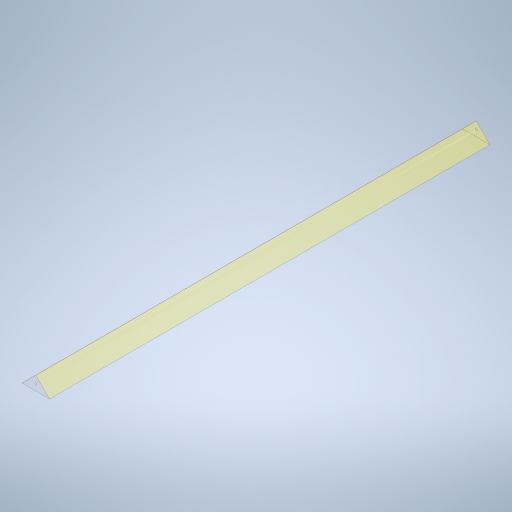
# Autodesk Inventor part: Centelladora triangular
Saved by Autodesk Inventor 2024.2 (Build 282272000, 272)
## iProperties
Created: 2024-08-22
Part Number: Centelladora triangular
Material: PMMA Plastic
Document SubType Name: Modeling
Designer: ja.restrepo1
Density: 1.188 g/cm^3
Appearance: Polycarbonate - Clear
Author: ja.restrepo1
Autodesk Inventor part; units mm, degrees
ref_plane "YZ Plane" through (0, 0, 0) normal (1, 0, 0) x (0, 1, 0)
ref_plane "XZ Plane" through (0, 0, 0) normal (0, 1, 0) x (-1, 0, 0)
ref_plane "XY Plane" through (0, 0, 0) normal (0, 0, 1) x (1, 0, 0)
sketch "Sketch1" plane through (0, 0, 0) normal (0, 0, 1) x (1, 0, 0)
  line L0 (19, 0) -> (-19, 0)
  line L1 (0, 0) -> (0, 19) construction
  line L2 (0, 19) -> (-19, 0)
  line L3 (0, 19) -> (19, 0)
  circle A0 centre (0, 8.7) radius 1.5
  dimension "d0" = 38
  dimension "d1" = 19
  dimension "d2" = 3
  dimension "d3" = 8.7
  constraints: 8 end point, 3 coincident, 1 centre point, 1 horizontal, 1 midpoint, 1 vertical, 1 vertical alignment, 2 other
  measures "d0" distance of L0.start L0.end
  measures "d1" distance of L1.start L1.end
  measures "d2" diameter of A0
  measures "d3" distance from line of A0.centre L0
extrude "centelladora triangular" add sketch "Sketch1" along normal mid plane 610
body "Solid1"
